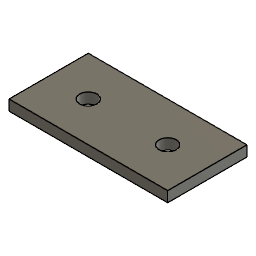
3030+Joining+Plate (Autodesk Fusion 360 design; units mm, degrees)
part number: 2026-02-08-17-44-25-026
Autodesk Fusion 360 part; units mm, degrees
note: some values were not read from the file. Set by a fixed rule: which sketch regions a step uses.
sketch "Sketch1" plane through (0, 0, 0) normal (0, 1, 0) x (1, 0, 0)
  line L0 (-59.6258, 37.8702) -> (0.3742, 37.8702)
  line L1 (0.3742, 37.8702) -> (0.3742, 7.8702)
  line L2 (0.3742, 7.8702) -> (-59.6258, 7.8702)
  line L3 (-59.6258, 7.8702) -> (-59.6258, 37.8702)
  circle A0 centre (-44.6258, 22.8702) radius 3.25
  circle A1 centre (-14.6258, 22.8702) radius 3.25
  line L4 (-44.6258, 37.8702) -> (-44.6258, 22.8702)
  line L5 (-59.6258, 22.8702) -> (-44.6258, 22.8702)
  line L6 (-44.6258, 22.8702) -> (-14.6258, 22.8702)
  point P0 (-32.4802, 26.6243)
  dimension "d1" = 60
  dimension "d2" = 30
  dimension "d3" = 6.5
  dimension "d4" = 6.5
  dimension "d5" = 15
  dimension "d6" = 15
  dimension "d7" = 30
  constraint horizontal L0
  constraint vertical L1
  constraint horizontal L2
  constraint vertical L3
  constraint vertical L4
  constraint coincident L0 L4.start
  constraint horizontal L5
  constraint coincident L3 L5.start
  constraint coincident A0.centre L4.end
  constraint perpendicular L4 L6
  constraint coincident A1.centre L6.end
  measures "d1" distance of L0.start L0.end
  measures "d2" distance of L0.start L2.end
  measures "d3" diameter of A0
  measures "d4" diameter of A1
  measures "d5" distance of L4.start A0.centre
  measures "d6" distance of L5.start A0.centre
  measures "d7" distance of A0.centre A1.centre
extrude "Extrude1" add sketch "Sketch1" along normal blind 4 contours L0 L3 A0 L4 L5 | L0 L1 L2 L3 A0 L4 L5
